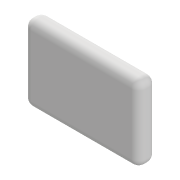
# Autodesk Inventor part: 00_Powerbank
Saved by Autodesk Inventor 2022 (Build 260153000, 153)
## iProperties
Created: 2022-04-02
Part Number: 00_Powerbank
Material: Generic
Document SubType Name: Modeling
Designer: Prakash Lab
Density: 1 g/cm^3
Appearance: Default
Author: Prakash Lab
Autodesk Inventor part; units mm, degrees
ref_plane "YZ Plane" through (0, 0, 0) normal (1, 0, 0) x (0, 1, 0)
ref_plane "XZ Plane" through (0, 0, 0) normal (0, 1, 0) x (-1, 0, 0)
ref_plane "XY Plane" through (0, 0, 0) normal (0, 0, 1) x (1, 0, 0)
sketch "Sketch1" plane through (0, 0, 0) normal (0, 0, 1) x (1, 0, 0)
  line L0 (46.5, 30.5) -> (-46.5, 30.5)
  line L1 (-46.5, 30.5) -> (-46.5, -30.5)
  line L2 (-46.5, -30.5) -> (46.5, -30.5)
  line L3 (46.5, -30.5) -> (46.5, 30.5)
  line L4 (46.5, 30.5) -> (-46.5, -30.5) construction
  line L5 (-46.5, 30.5) -> (46.5, -30.5) construction
  point P0 (0, 0)
  dimension "d0" = 93
  dimension "d1" = 61
  constraints: 12 end point, 2 midpoint, 2 parallel, 1 horizontal, 1 perpendicular
  measures "d0" distance of L0.start L0.end
  measures "d1" distance of L1.end L0.end
extrude "Extrusion1" add sketch "Sketch1" along normal blind 14.4
fillet "Fillet1" radius 6 12 edges at (46.5, 30.5, 7.2) (-46.5, 30.5, 7.2) (46.5, -30.5, 7.2) (-46.5, -30.5, 7.2) (0, 30.5, 14.4) (0, 30.5, 0) (46.5, 0, 0) (46.5, 0, 14.4) (0, -30.5, 14.4) (0, -30.5, 0) (-46.5, 0, 14.4) (-46.5, 0, 0)
body "Solid1"
